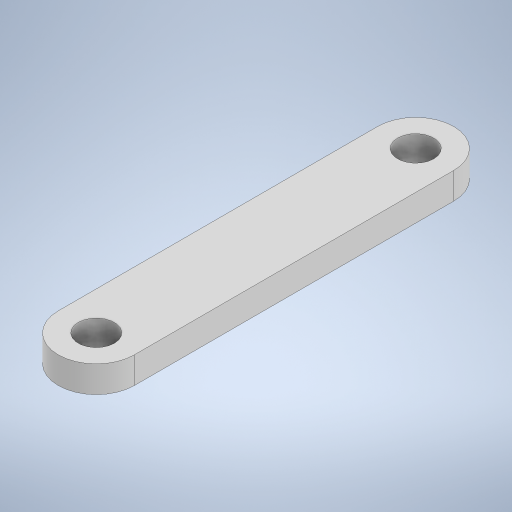
# Autodesk Inventor part: Linear Arm
Saved by Autodesk Inventor 2024 (Build 280153000, 153)
## iProperties
Created: 2023-04-23
Part Number: Linear Arm
Material: Generic
Document SubType Name: Modeling
Designer: byrne
Density: 1 g/cm^3
Appearance: Default
Author: byrne
Autodesk Inventor part; units mm, degrees
ref_plane "YZ Plane" through (0, 0, 0) normal (1, 0, 0) x (0, 1, 0)
ref_plane "XZ Plane" through (0, 0, 0) normal (0, 1, 0) x (-1, 0, 0)
ref_plane "XY Plane" through (0, 0, 0) normal (0, 0, 1) x (1, 0, 0)
sketch "Sketch1" plane through (0, 0, 0) normal (0, 1, 0) x (-1, 0, 0)
  circle A0 centre (0, 0) radius 2.159
  circle A1 centre (0, 38.1) radius 2.159
  circle A2 centre (0, 38.1) radius 4.5403
  circle A3 centre (0, 0) radius 4.5403
  line L0 (4.5403, 38.1) -> (4.5402, 0)
  line L1 (-4.5403, 0) -> (-4.5403, 38.1)
  dimension "d0" = 4.318
  dimension "d1" = 4.318
  dimension "d2" = 38.1
  dimension "d3" = 2.3813
  dimension "d4" = 2.3813
  constraints: 4 centre point, 4 end point, 4 point on circle, 4 tangent, 1 coincident, 1 vertical alignment
  measures "d0" diameter of A0
  measures "d1" diameter of A1
  measures "d2" distance of A0.centre A1.centre
  measures "d3" radial gap between concentric circles of A1 A2
  measures "d4" radial gap between concentric circles of A0 A3
extrude "Extrusion1" add sketch "Sketch1" along normal blind 3.175
body "Solid1"
